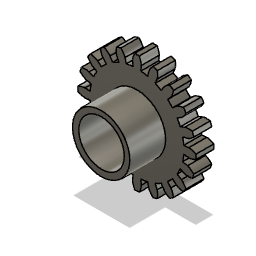
assembly (Autodesk Fusion 360 archive; units mm, degrees)
design "Small Gear(30mm)"
Autodesk Fusion 360 part; units mm, degrees
sketch "Sketch1" plane through (0, 0, 0) normal (0, 0, 1) x (1, 0, 0)
  spline S0 degree 5 poles (14.4718, -1.2197) (14.4719, -1.2197) (14.4721, -1.2197) (14.4724, -1.2198) (14.473, -1.2198) (14.4738, -1.2199) (14.4747, -1.2199) (14.4757, -1.22) (14.4769, -1.22) (14.4781, -1.2201) (14.4795, -1.2202) (14.481, -1.2203) (14.4826, -1.2203) (14.4844, -1.2204) (14.4862, -1.2205) (14.4881, -1.2205) (14.4902, -1.2206) (14.4923, -1.2207) (14.4946, -1.2207) (14.497, -1.2208) (14.4994, -1.2209) (14.502, -1.2209) (14.5047, -1.221) (14.5074, -1.221) (14.5103, -1.221) (14.5133, -1.2211) (14.5163, -1.2211) (14.5195, -1.2211) (14.5227, -1.2211) (14.5261, -1.2211) (14.5295, -1.2211) (14.533, -1.2211) (14.5366, -1.221) (14.5403, -1.221) (14.5441, -1.2209) (14.548, -1.2208) (14.5519, -1.2208) (14.556, -1.2207) (14.5601, -1.2206) (14.5643, -1.2204) (14.5686, -1.2203) (14.573, -1.2202) (14.5775, -1.22) (14.582, -1.2198) (14.5866, -1.2196) (14.5913, -1.2194) (14.5961, -1.2192) (14.601, -1.219) (14.6059, -1.2187) (14.6109, -1.2185) (14.616, -1.2182) (14.6212, -1.2179) (14.6264, -1.2176) (14.6317, -1.2172) (14.6371, -1.2169) (14.6425, -1.2165) (14.648, -1.2161) (14.6536, -1.2157) (14.6593, -1.2153) (14.665, -1.2148) (14.6708, -1.2143) (14.6767, -1.2139) (14.6827, -1.2133) (14.6887, -1.2128) (14.6947, -1.2123) (14.7009, -1.2117) (14.7071, -1.2111) (14.7133, -1.2105) (14.7197, -1.2098) (14.7261, -1.2092) (14.7325, -1.2085) (14.7391, -1.2078) (14.7457, -1.2071) (14.7523, -1.2063) (14.759, -1.2056) (14.7658, -1.2048) (14.7726, -1.204) (14.7795, -1.2031) (14.7865, -1.2023) (14.7935, -1.2014) (14.8006, -1.2005) (14.8077, -1.1995) (14.8149, -1.1986) (14.8221, -1.1976) (14.8294, -1.1966) (14.8368, -1.1955) (14.8442, -1.1945) (14.8517, -1.1934) (14.8592, -1.1923) (14.8668, -1.1911) (14.8744, -1.19) (14.8821, -1.1888) (14.8899, -1.1876) (14.8977, -1.1863) (14.9055, -1.1851) (14.9134, -1.1838) (14.9214, -1.1825) (14.9294, -1.1811) (14.9375, -1.1797) (14.9456, -1.1783) (14.9537, -1.1769) (14.9619, -1.1754) (14.9702, -1.174) (14.9785, -1.1724) (14.9869, -1.1709) (14.9953, -1.1693) (15.0037, -1.1677) (15.0122, -1.1661) (15.0208, -1.1645) (15.0294, -1.1628) (15.038, -1.1611) (15.0467, -1.1593) (15.0555, -1.1576) (15.0643, -1.1558) (15.0731, -1.1539) (15.082, -1.1521) (15.0909, -1.1502) (15.0999, -1.1483) (15.1089, -1.1463) (15.1179, -1.1444) (15.127, -1.1423) (15.1362, -1.1403) (15.1454, -1.1382) (15.1546, -1.1361) (15.1639, -1.134) (15.1732, -1.1319) (15.1825, -1.1297) (15.1919, -1.1275) (15.2014, -1.1252) (15.2109, -1.1229) (15.2204, -1.1206) (15.2299, -1.1183) (15.2395, -1.1159) (15.2492, -1.1135) (15.2589, -1.1111) (15.2686, -1.1086) (15.2783, -1.1061) (15.2881, -1.1036) (15.298, -1.101) (15.3079, -1.0984) (15.3178, -1.0958) (15.3277, -1.0931) (15.3377, -1.0905) (15.3477, -1.0877) (15.3578, -1.085) (15.3679, -1.0822) (15.3781, -1.0794) (15.3882, -1.0765) (15.3984, -1.0737) (15.4087, -1.0707) (15.419, -1.0678) (15.4293, -1.0648) (15.4396, -1.0618) (15.45, -1.0587) (15.4604, -1.0557) (15.4709, -1.0526) (15.4814, -1.0494) (15.4919, -1.0462) (15.5025, -1.043) (15.513, -1.0398) (15.5237, -1.0365) (15.5343, -1.0332) (15.545, -1.0298) (15.5557, -1.0265) (15.5665, -1.0231) (15.5773, -1.0196) (15.5881, -1.0161) (15.5989, -1.0126) (15.6098, -1.0091) (15.6207, -1.0055) (15.6317, -1.0019) (15.6426, -0.9982) (15.6536, -0.9945) (15.6647, -0.9908) (15.6757, -0.9871) (15.6868, -0.9833) (15.6979, -0.9795) (15.7091, -0.9756) (15.7203, -0.9717) (15.7315, -0.9678) (15.7427, -0.9638) (15.754, -0.9598) (15.7653, -0.9558) (15.7766, -0.9518) (15.7879, -0.9477) (15.7993, -0.9435) (15.8107, -0.9394) (15.8222, -0.9352) (15.8336, -0.9309) (15.8451, -0.9267) (15.8566, -0.9223) (15.8681, -0.918) (15.8797, -0.9136) (15.8913, -0.9092) (15.9029, -0.9048) (15.9146, -0.9003) (15.9262, -0.8958) (15.9379, -0.8912) (15.9496, -0.8866) (15.9614, -0.882) (15.9731, -0.8773) (15.9849, -0.8727) (15.9967, -0.8679) (16.0086, -0.8632) (16.0205, -0.8584) (16.0323, -0.8535) (16.0442, -0.8487) (16.0562, -0.8437) (16.0681, -0.8388) (16.0801, -0.8338) (16.0921, -0.8288) (16.1041, -0.8238) (16.1162, -0.8187) (16.1283, -0.8135) (16.1404, -0.8084) (16.1525, -0.8032) (16.1646, -0.798) (16.1768, -0.7927) (16.1889, -0.7874) (16.2011, -0.7821) (16.2134, -0.7767) (16.2256, -0.7713) (16.2379, -0.7658) (16.2502, -0.7603) (16.2625, -0.7548) (16.2748, -0.7493) (16.2871, -0.7437) (16.2995, -0.738) (16.3119, -0.7324) (16.3243, -0.7267) (16.3367, -0.7209) (16.3491, -0.7152) (16.3616, -0.7094) (16.3741, -0.7035) (16.3866, -0.6976) (16.3991, -0.6917) (16.4116, -0.6858) (16.4242, -0.6798) (16.4368, -0.6737) (16.4493, -0.6677) (16.4619, -0.6616) (16.472, -0.6567) (16.4796, -0.653) (16.4847, -0.6505) (16.4872, -0.6492) knots 0 0 0 0 0 0 0.00416667 0.00833333 0.0125 0.01666667 0.02083333 0.025 0.02916667 0.03333333 0.0375 0.04166667 0.04583333 0.05 0.05416667 0.05833333 0.0625 0.06666667 0.07083333 0.075 0.07916667 0.08333333 0.0875 0.09166667 0.09583333 0.1 0.10416667 0.10833333 0.1125 0.11666667 0.12083333 0.125 0.12916667 0.13333333 0.1375 0.14166667 0.14583333 0.15 0.15416667 0.15833333 0.1625 0.16666667 0.17083333 0.175 0.17916667 0.18333333 0.1875 0.19166667 0.19583333 0.2 0.20416667 0.20833333 0.2125 0.21666667 0.22083333 0.225 0.22916667 0.23333333 0.2375 0.24166667 0.24583333 0.25 0.25416667 0.25833333 0.2625 0.26666667 0.27083333 0.275 0.27916667 0.28333333 0.2875 0.29166667 0.29583333 0.3 0.30416667 0.30833333 0.3125 0.31666667 0.32083333 0.325 0.32916667 0.33333333 0.3375 0.34166667 0.34583333 0.35 0.35416667 0.35833333 0.3625 0.36666667 0.37083333 0.375 0.37916667 0.38333333 0.3875 0.39166667 0.39583333 0.4 0.40416667 0.40833333 0.4125 0.41666667 0.42083333 0.425 0.42916667 0.43333333 0.4375 0.44166667 0.44583333 0.45 0.45416667 0.45833333 0.4625 0.46666667 0.47083333 0.475 0.47916667 0.48333333 0.4875 0.49166667 0.49583333 0.5 0.50416667 0.50833333 0.5125 0.51666667 0.52083333 0.525 0.52916667 0.53333333 0.5375 0.54166667 0.54583333 0.55 0.55416667 0.55833333 0.5625 0.56666667 0.57083333 0.575 0.57916667 0.58333333 0.5875 0.59166667 0.59583333 0.6 0.60416667 0.60833333 0.6125 0.61666667 0.62083333 0.625 0.62916667 0.63333333 0.6375 0.64166667 0.64583333 0.65 0.65416667 0.65833333 0.6625 0.66666667 0.67083333 0.675 0.67916667 0.68333333 0.6875 0.69166667 0.69583333 0.7 0.70416667 0.70833333 0.7125 0.71666667 0.72083333 0.725 0.72916667 0.73333333 0.7375 0.74166667 0.74583333 0.75 0.75416667 0.75833333 0.7625 0.76666667 0.77083333 0.775 0.77916667 0.78333333 0.7875 0.79166667 0.79583333 0.8 0.80416667 0.80833333 0.8125 0.81666667 0.82083333 0.825 0.82916667 0.83333333 0.8375 0.84166667 0.84583333 0.85 0.85416667 0.85833333 0.8625 0.86666667 0.87083333 0.875 0.87916667 0.88333333 0.8875 0.89166667 0.89583333 0.9 0.90416667 0.90833333 0.9125 0.91666667 0.92083333 0.925 0.92916667 0.93333333 0.9375 0.94166667 0.94583333 0.95 0.95416667 0.95833333 0.9625 0.96666667 0.97083333 0.975 0.97916667 0.98333333 0.9875 0.99166667 0.99583333 1 1 1 1 1 1
  spline S1 degree 5 poles (14.4718, 1.2197) (14.4719, 1.2197) (14.4721, 1.2197) (14.4724, 1.2198) (14.473, 1.2198) (14.4738, 1.2199) (14.4747, 1.2199) (14.4757, 1.22) (14.4769, 1.22) (14.4781, 1.2201) (14.4795, 1.2202) (14.481, 1.2203) (14.4826, 1.2203) (14.4844, 1.2204) (14.4862, 1.2205) (14.4881, 1.2205) (14.4902, 1.2206) (14.4923, 1.2207) (14.4946, 1.2207) (14.497, 1.2208) (14.4994, 1.2209) (14.502, 1.2209) (14.5047, 1.221) (14.5074, 1.221) (14.5103, 1.221) (14.5133, 1.2211) (14.5163, 1.2211) (14.5195, 1.2211) (14.5227, 1.2211) (14.5261, 1.2211) (14.5295, 1.2211) (14.533, 1.2211) (14.5366, 1.221) (14.5403, 1.221) (14.5441, 1.2209) (14.548, 1.2208) (14.5519, 1.2208) (14.556, 1.2207) (14.5601, 1.2206) (14.5643, 1.2204) (14.5686, 1.2203) (14.573, 1.2202) (14.5775, 1.22) (14.582, 1.2198) (14.5866, 1.2196) (14.5913, 1.2194) (14.5961, 1.2192) (14.601, 1.219) (14.6059, 1.2187) (14.6109, 1.2185) (14.616, 1.2182) (14.6212, 1.2179) (14.6264, 1.2176) (14.6317, 1.2172) (14.6371, 1.2169) (14.6425, 1.2165) (14.648, 1.2161) (14.6536, 1.2157) (14.6593, 1.2153) (14.665, 1.2148) (14.6708, 1.2143) (14.6767, 1.2139) (14.6827, 1.2133) (14.6887, 1.2128) (14.6947, 1.2123) (14.7009, 1.2117) (14.7071, 1.2111) (14.7133, 1.2105) (14.7197, 1.2098) (14.7261, 1.2092) (14.7325, 1.2085) (14.7391, 1.2078) (14.7457, 1.2071) (14.7523, 1.2063) (14.759, 1.2056) (14.7658, 1.2048) (14.7726, 1.204) (14.7795, 1.2031) (14.7865, 1.2023) (14.7935, 1.2014) (14.8006, 1.2005) (14.8077, 1.1995) (14.8149, 1.1986) (14.8221, 1.1976) (14.8294, 1.1966) (14.8368, 1.1955) (14.8442, 1.1945) (14.8517, 1.1934) (14.8592, 1.1923) (14.8668, 1.1911) (14.8744, 1.19) (14.8821, 1.1888) (14.8899, 1.1876) (14.8977, 1.1863) (14.9055, 1.1851) (14.9134, 1.1838) (14.9214, 1.1825) (14.9294, 1.1811) (14.9375, 1.1797) (14.9456, 1.1783) (14.9537, 1.1769) (14.9619, 1.1754) (14.9702, 1.174) (14.9785, 1.1724) (14.9869, 1.1709) (14.9953, 1.1693) (15.0037, 1.1677) (15.0122, 1.1661) (15.0208, 1.1645) (15.0294, 1.1628) (15.038, 1.1611) (15.0467, 1.1593) (15.0555, 1.1576) (15.0643, 1.1558) (15.0731, 1.1539) (15.082, 1.1521) (15.0909, 1.1502) (15.0999, 1.1483) (15.1089, 1.1463) (15.1179, 1.1444) (15.127, 1.1423) (15.1362, 1.1403) (15.1454, 1.1382) (15.1546, 1.1361) (15.1639, 1.134) (15.1732, 1.1319) (15.1825, 1.1297) (15.1919, 1.1275) (15.2014, 1.1252) (15.2109, 1.1229) (15.2204, 1.1206) (15.2299, 1.1183) (15.2395, 1.1159) (15.2492, 1.1135) (15.2589, 1.1111) (15.2686, 1.1086) (15.2783, 1.1061) (15.2881, 1.1036) (15.298, 1.101) (15.3079, 1.0984) (15.3178, 1.0958) (15.3277, 1.0931) (15.3377, 1.0905) (15.3477, 1.0877) (15.3578, 1.085) (15.3679, 1.0822) (15.3781, 1.0794) (15.3882, 1.0765) (15.3984, 1.0737) (15.4087, 1.0707) (15.419, 1.0678) (15.4293, 1.0648) (15.4396, 1.0618) (15.45, 1.0587) (15.4604, 1.0557) (15.4709, 1.0526) (15.4814, 1.0494) (15.4919, 1.0462) (15.5025, 1.043) (15.513, 1.0398) (15.5237, 1.0365) (15.5343, 1.0332) (15.545, 1.0298) (15.5557, 1.0265) (15.5665, 1.0231) (15.5773, 1.0196) (15.5881, 1.0161) (15.5989, 1.0126) (15.6098, 1.0091) (15.6207, 1.0055) (15.6317, 1.0019) (15.6426, 0.9982) (15.6536, 0.9945) (15.6647, 0.9908) (15.6757, 0.9871) (15.6868, 0.9833) (15.6979, 0.9795) (15.7091, 0.9756) (15.7203, 0.9717) (15.7315, 0.9678) (15.7427, 0.9638) (15.754, 0.9598) (15.7653, 0.9558) (15.7766, 0.9518) (15.7879, 0.9477) (15.7993, 0.9435) (15.8107, 0.9394) (15.8222, 0.9352) (15.8336, 0.9309) (15.8451, 0.9267) (15.8566, 0.9223) (15.8681, 0.918) (15.8797, 0.9136) (15.8913, 0.9092) (15.9029, 0.9048) (15.9146, 0.9003) (15.9262, 0.8958) (15.9379, 0.8912) (15.9496, 0.8866) (15.9614, 0.882) (15.9731, 0.8773) (15.9849, 0.8727) (15.9967, 0.8679) (16.0086, 0.8632) (16.0205, 0.8584) (16.0323, 0.8535) (16.0442, 0.8487) (16.0562, 0.8437) (16.0681, 0.8388) (16.0801, 0.8338) (16.0921, 0.8288) (16.1041, 0.8238) (16.1162, 0.8187) (16.1283, 0.8135) (16.1404, 0.8084) (16.1525, 0.8032) (16.1646, 0.798) (16.1768, 0.7927) (16.1889, 0.7874) (16.2011, 0.7821) (16.2134, 0.7767) (16.2256, 0.7713) (16.2379, 0.7658) (16.2502, 0.7603) (16.2625, 0.7548) (16.2748, 0.7493) (16.2871, 0.7437) (16.2995, 0.738) (16.3119, 0.7324) (16.3243, 0.7267) (16.3367, 0.7209) (16.3491, 0.7152) (16.3616, 0.7094) (16.3741, 0.7035) (16.3866, 0.6976) (16.3991, 0.6917) (16.4116, 0.6858) (16.4242, 0.6798) (16.4368, 0.6737) (16.4493, 0.6677) (16.4619, 0.6616) (16.472, 0.6567) (16.4796, 0.653) (16.4847, 0.6505) (16.4872, 0.6492) knots 0 0 0 0 0 0 0.00416667 0.00833333 0.0125 0.01666667 0.02083333 0.025 0.02916667 0.03333333 0.0375 0.04166667 0.04583333 0.05 0.05416667 0.05833333 0.0625 0.06666667 0.07083333 0.075 0.07916667 0.08333333 0.0875 0.09166667 0.09583333 0.1 0.10416667 0.10833333 0.1125 0.11666667 0.12083333 0.125 0.12916667 0.13333333 0.1375 0.14166667 0.14583333 0.15 0.15416667 0.15833333 0.1625 0.16666667 0.17083333 0.175 0.17916667 0.18333333 0.1875 0.19166667 0.19583333 0.2 0.20416667 0.20833333 0.2125 0.21666667 0.22083333 0.225 0.22916667 0.23333333 0.2375 0.24166667 0.24583333 0.25 0.25416667 0.25833333 0.2625 0.26666667 0.27083333 0.275 0.27916667 0.28333333 0.2875 0.29166667 0.29583333 0.3 0.30416667 0.30833333 0.3125 0.31666667 0.32083333 0.325 0.32916667 0.33333333 0.3375 0.34166667 0.34583333 0.35 0.35416667 0.35833333 0.3625 0.36666667 0.37083333 0.375 0.37916667 0.38333333 0.3875 0.39166667 0.39583333 0.4 0.40416667 0.40833333 0.4125 0.41666667 0.42083333 0.425 0.42916667 0.43333333 0.4375 0.44166667 0.44583333 0.45 0.45416667 0.45833333 0.4625 0.46666667 0.47083333 0.475 0.47916667 0.48333333 0.4875 0.49166667 0.49583333 0.5 0.50416667 0.50833333 0.5125 0.51666667 0.52083333 0.525 0.52916667 0.53333333 0.5375 0.54166667 0.54583333 0.55 0.55416667 0.55833333 0.5625 0.56666667 0.57083333 0.575 0.57916667 0.58333333 0.5875 0.59166667 0.59583333 0.6 0.60416667 0.60833333 0.6125 0.61666667 0.62083333 0.625 0.62916667 0.63333333 0.6375 0.64166667 0.64583333 0.65 0.65416667 0.65833333 0.6625 0.66666667 0.67083333 0.675 0.67916667 0.68333333 0.6875 0.69166667 0.69583333 0.7 0.70416667 0.70833333 0.7125 0.71666667 0.72083333 0.725 0.72916667 0.73333333 0.7375 0.74166667 0.74583333 0.75 0.75416667 0.75833333 0.7625 0.76666667 0.77083333 0.775 0.77916667 0.78333333 0.7875 0.79166667 0.79583333 0.8 0.80416667 0.80833333 0.8125 0.81666667 0.82083333 0.825 0.82916667 0.83333333 0.8375 0.84166667 0.84583333 0.85 0.85416667 0.85833333 0.8625 0.86666667 0.87083333 0.875 0.87916667 0.88333333 0.8875 0.89166667 0.89583333 0.9 0.90416667 0.90833333 0.9125 0.91666667 0.92083333 0.925 0.92916667 0.93333333 0.9375 0.94166667 0.94583333 0.95 0.95416667 0.95833333 0.9625 0.96666667 0.97083333 0.975 0.97916667 0.98333333 0.9875 0.99166667 0.99583333 1 1 1 1 1 1
  spline S2 degree 5 poles (14.4709, -1.2197) (14.4709, -1.2197) (14.471, -1.2197) (14.4711, -1.2197) (14.4713, -1.2197) (14.4714, -1.2197) (14.4716, -1.2197) (14.4717, -1.2197) (14.4717, -1.2197) (14.4718, -1.2197) knots 0 0 0 0 0 0 0.2 0.4 0.6 0.8 1 1 1 1 1 1
  spline S3 degree 5 poles (14.4709, 1.2197) (14.4709, 1.2197) (14.471, 1.2197) (14.4711, 1.2197) (14.4713, 1.2197) (14.4714, 1.2197) (14.4716, 1.2197) (14.4717, 1.2197) (14.4717, 1.2197) (14.4718, 1.2197) knots 0 0 0 0 0 0 0.2 0.4 0.6 0.8 1 1 1 1 1 1
  line L0 (0, 0) -> (14.4709, -1.2197)
  line L1 (0, 0) -> (14.4709, 1.2197)
  arc A0 (16.4872, -0.6492) -> (16.4872, 0.6492) centre (0, 0) ccw
  point P0 (14.4744, -1.2199)
  point P1 (14.4788, -1.2201)
  point P2 (14.485, -1.2204)
  point P3 (14.4929, -1.2207)
  point P4 (14.5026, -1.2209)
  point P5 (14.514, -1.2211)
  point P6 (14.5272, -1.2211)
  point P7 (14.5421, -1.2209)
  point P8 (14.5589, -1.2206)
  point P9 (14.5773, -1.22)
  point P10 (14.5975, -1.2192)
  point P11 (14.6195, -1.218)
  point P12 (14.6432, -1.2164)
  point P13 (14.6687, -1.2145)
  point P14 (14.6958, -1.2122)
  point P15 (14.7247, -1.2093)
  point P16 (14.7553, -1.206)
  point P17 (14.7877, -1.2021)
  point P18 (14.8217, -1.1976)
  point P19 (14.8574, -1.1925)
  point P20 (14.8948, -1.1868)
  point P21 (14.9338, -1.1803)
  point P22 (14.9746, -1.1732)
  point P23 (15.0169, -1.1652)
  point P24 (15.0609, -1.1564)
  point P25 (15.1066, -1.1468)
  point P26 (15.1538, -1.1363)
  point P27 (15.2026, -1.1249)
  point P28 (15.2531, -1.1125)
  point P29 (15.305, -1.0992)
  point P30 (15.3586, -1.0848)
  point P31 (15.4136, -1.0693)
  point P32 (15.4702, -1.0528)
  point P33 (15.5283, -1.0351)
  point P34 (15.5878, -1.0162)
  point P35 (15.6488, -0.9961)
  point P36 (15.7113, -0.9748)
  point P37 (15.7752, -0.9523)
  point P38 (15.8404, -0.9284)
  point P39 (15.9071, -0.9032)
  point P40 (15.9751, -0.8766)
  point P41 (16.0444, -0.8486)
  point P42 (16.1151, -0.8191)
  point P43 (16.187, -0.7882)
  point P44 (16.2603, -0.7558)
  point P45 (16.3347, -0.7219)
  point P46 (16.4104, -0.6863)
  point P47 (14.4744, 1.2199)
  point P48 (14.4788, 1.2201)
  point P49 (14.485, 1.2204)
  point P50 (14.4929, 1.2207)
  point P51 (14.5026, 1.2209)
  point P52 (14.514, 1.2211)
  point P53 (14.5272, 1.2211)
  point P54 (14.5421, 1.2209)
  point P55 (14.5589, 1.2206)
  point P56 (14.5773, 1.22)
  point P57 (14.5975, 1.2192)
  point P58 (14.6195, 1.218)
  point P59 (14.6432, 1.2164)
  point P60 (14.6687, 1.2145)
  point P61 (14.6958, 1.2122)
  point P62 (14.7247, 1.2093)
  point P63 (14.7553, 1.206)
  point P64 (14.7877, 1.2021)
  point P65 (14.8217, 1.1976)
  point P66 (14.8574, 1.1925)
  point P67 (14.8948, 1.1868)
  point P68 (14.9338, 1.1803)
  point P69 (14.9746, 1.1732)
  point P70 (15.0169, 1.1652)
  point P71 (15.0609, 1.1564)
  point P72 (15.1066, 1.1468)
  point P73 (15.1538, 1.1363)
  point P74 (15.2026, 1.1249)
  point P75 (15.2531, 1.1125)
  point P76 (15.305, 1.0992)
  point P77 (15.3586, 1.0848)
  point P78 (15.4136, 1.0693)
  point P79 (15.4702, 1.0528)
  point P80 (15.5283, 1.0351)
  point P81 (15.5878, 1.0162)
  point P82 (15.6488, 0.9961)
  point P83 (15.7113, 0.9748)
  point P84 (15.7752, 0.9523)
  point P85 (15.8404, 0.9284)
  point P86 (15.9071, 0.9032)
  point P87 (15.9751, 0.8766)
  point P88 (16.0444, 0.8486)
  point P89 (16.1151, 0.8191)
  point P90 (16.187, 0.7882)
  point P91 (16.2603, 0.7558)
  point P92 (16.3347, 0.7219)
  point P93 (16.4104, 0.6863)
sketch "Sketch2" plane through (0, 0, 0) normal (0, 0, 1) x (1, 0, 0)
  circle A0 centre (0, 0) radius 13.125
extrude "Extrude1" add sketch "Sketch2" along normal blind 5 makes body 1
extrude "Extrude2" add sketch "Sketch1" along normal blind 5 separate body makes body 2
pattern_circular "C-Pattern1" count 20 over 360 about axis through (0, 0, 1.75) along (0, 0, 1) of "Extrude2" makes body 3 at (4.7135, 1.104, 1.6667) makes body 4 at (4.1416, 2.5065, 1.6667) makes body 5 at (3.1644, 3.6637, 1.6667) makes body 6 at (1.8774, 4.4622, 1.6667) makes body 7 at (0.4066, 4.8239, 1.6667) makes body 8 at (-1.104, 4.7135, 1.6667) makes body 9 at (-3.1644, 3.6637, 1.6667) makes body 10 at (-3.6637, 3.1644, 1.6667) makes body 11 at (-4.7135, 1.104, 1.6667) makes body 12 at (-4.8239, 0.4066, 1.6667) makes body 13 at (-4.7135, -1.104, 1.6667) makes body 14 at (-3.6637, -3.1644, 1.6667) makes body 15 at (-3.1644, -3.6637, 1.6667) makes body 16 at (-1.8774, -4.4622, 1.6667) makes body 17 at (-0.4066, -4.8239, 1.6667) makes body 18 at (1.104, -4.7135, 1.6667) makes body 19 at (2.5065, -4.1416, 1.6667) makes body 20 at (3.6637, -3.1644, 1.6667) makes body 21 at (4.4622, -1.8774, 1.6667)
combine "Combine1" operation add target body 1 tool bodies 2 3 4 5 6 7 8 9 10 11 12 13 14 15 16 17 18 19 20 21
sketch "Sketch3" plane through (0, 0, 0) normal (0, 0, 1) x (1, 0, 0)
  line L0 (0, 0) -> (48.3003, 0) construction
  line L1 (48.3003, 0) -> (48.3003, 3) construction
  line L2 (48.3003, 3) -> (0, 3) construction
  line L3 (0, 3) -> (0, 0) construction
  constraint perpendicular L0 L1
  constraint parallel L0 L2
  constraint parallel L1 L3
cylinder "CylinderPrimitive1" add diameter 16 height 10 placed x (1, 0, 0) y (0, 1, 0) z (0, 0, 1) at (0, 0, 5) bodies 1
hole "Hole1" at (0.103, 0.1545, 15) direction (0, 0, -1) diameter 12.7 depth 30 tip angle 118 bodies 1

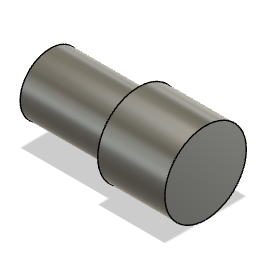
design "motor finale"
Autodesk Fusion 360 part; units mm, degrees
cylinder "CylinderPrimitive1" add diameter 37 height 30.5 placed x (0, 0, -1) y (0, 1, 0) z (1, 0, 0) at (0, 0, 0)
cylinder "CylinderPrimitive2" add diameter 27.5 height 40 placed x (0, 0, 1) y (0, 1, 0) z (-1, 0, 0) at (0, 0, 0)

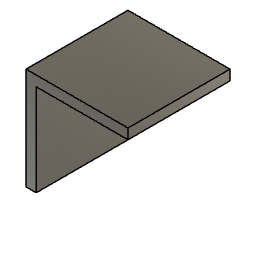
design "L_Support"
Autodesk Fusion 360 part; units mm, degrees
sketch "Sketch1" plane through (0, 0, 0) normal (0, 1, 0) x (1, 0, 0)
  line L0 (0, 0) -> (5, 0)
  line L1 (5, 0) -> (5, -50)
  line L2 (5, -50) -> (0, -50)
  line L3 (0, -50) -> (0, 0)
  line L4 (0, -50) -> (50, -50)
  line L5 (50, -50) -> (50, -45)
  line L6 (50, -45) -> (0, -45)
  line L7 (0, -45) -> (0, -50)
  dimension "d1" = 5
  dimension "d2" = 50
  dimension "d3" = 50
  dimension "d4" = 5
  constraint horizontal L0
  constraint vertical L1
  constraint horizontal L2
  constraint vertical L3
  constraint coincident L0.start L3.end
  constraint horizontal L4
  constraint vertical L5
  constraint horizontal L6
  constraint vertical L7
  measures "d1" distance of L0.start L0.end
  measures "d2" distance of L0.start L2.end
  measures "d3" distance of L2.end L4.end
  measures "d4" distance of L2.end L6.end
extrude "Extrude1" add sketch "Sketch1" along normal blind 50

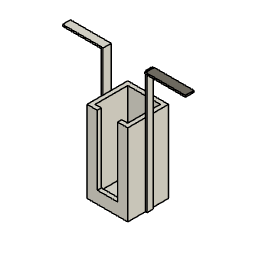
design "Container Seed"
Autodesk Fusion 360 part; units mm, degrees
sketch "Sketch1" plane through (0, 0, 0) normal (0, 0, 1) x (1, 0, 0)
  line L0 (0, 0) -> (50, 0)
  line L1 (50, 0) -> (50, 50)
  line L2 (50, 50) -> (0, 50)
  line L3 (0, 50) -> (0, 0)
  line L4 (5, 5) -> (45, 5)
  line L5 (45, 5) -> (45, 45)
  line L6 (45, 45) -> (5, 45)
  line L7 (5, 45) -> (5, 5)
  dimension "d1" = 50
  dimension "d2" = 50
  dimension "d3" = 40
  constraint horizontal L0
  constraint vertical L1
  constraint horizontal L2
  constraint vertical L3
  constraint coincident L0.start L3.end
  constraint horizontal L4
  constraint vertical L5
  constraint horizontal L6
  constraint vertical L7
  measures "d1" distance of L0.start L0.end
  measures "d2" distance of L0.start L2.end
  measures "d3" distance of L4.start L4.end
extrude "Extrude1" add sketch "Sketch1" along normal blind 95 makes body 1
sketch "Sketch2" plane through (0, 0, 0) normal (0, 0, 1) x (1, 0, 0)
  line L0 (0, 0) -> (50, 0)
  line L1 (50, 0) -> (50, 50)
  line L2 (50, 50) -> (0, 50)
  line L3 (0, 50) -> (0, 0)
  constraint horizontal L0
  constraint vertical L1
  constraint horizontal L2
  constraint vertical L3
  constraint coincident L0.start L3.end
extrude "Extrude2" add sketch "Sketch2" against normal blind 5 bodies 1
sketch "Sketch3" plane through (0, 0, 0) normal (0, 1, 0) x (1, 0, 0)
  line L0 (25, -95) -> (12.5, -95)
  line L1 (12.5, -95) -> (12.5, -30)
  line L2 (12.5, -30) -> (25, -30)
  line L3 (25, -30) -> (25, -95)
  dimension "d8" = 12.5
  dimension "d9" = 65
  constraint horizontal L0
  constraint vertical L1
  constraint horizontal L2
  constraint vertical L3
  measures "d8" distance of L0.start L0.end
  measures "d9" distance of L0.start L2.end
sketch "Sketch4" plane through (0, 0, 0) normal (0, 1, 0) x (1, 0, 0)
  line L0 (25, -30) -> (37.5, -30)
  line L1 (37.5, -30) -> (37.5, -95)
  line L2 (37.5, -95) -> (25, -95)
  line L3 (25, -95) -> (25, -30)
  dimension "d10" = 12.5
  dimension "d11" = 65
  constraint horizontal L0
  constraint vertical L1
  constraint horizontal L2
  constraint vertical L3
  measures "d10" distance of L0.start L0.end
  measures "d11" distance of L0.start L2.end
extrude "Extrude3" cut sketch "Sketch3" along normal blind 20 bodies 1
extrude "Extrude4" cut sketch "Sketch4" along normal blind 10 bodies 1
extrude "Extrude5" cut 1 faces at (20.8333, 1.6667, 30) along direction (0, 0, -1) blind 20 on bodies 1 bodies 1
box "BoxPrimitive1" add length 150 width 7.6164 height 2 placed x (0, 0, 1) y (0, -1, 0) z (1, 0, 0) at (50, 29.2955, -5) bodies 1
box "BoxPrimitive2" add length 150 width 10.3045 height 2 placed x (0, 0, 1) y (0, 1, 0) z (-1, 0, 0) at (0, 19.439, -5) bodies 1
box "BoxPrimitive3" add length 2 width 9.6811 height -50 placed x (0, 0, 1) y (0, -1, 0) z (1, 0, 0) at (0, 29.6811, 143) bodies 1
box "BoxPrimitive4" add length 2 width 10.4962 height 50 placed x (0, 0, 1) y (0, -1, 0) z (1, 0, 0) at (0, -89.5038, 150) separate body makes body 2
move_body "Move1" bodies 2 to x (1, 0, 0) y (0, 1, 0) z (0, 0, 1) at (50.5817, 120.1851, -7.2633)

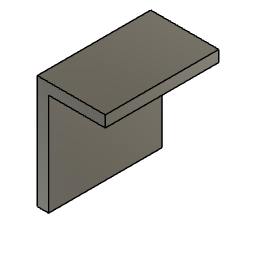
design "Motor Mount"
Autodesk Fusion 360 part; units mm, degrees
sketch "Sketch1" plane through (0, 0, 0) normal (0, 1, 0) x (1, 0, 0)
  line L0 (0, 0) -> (5, 0)
  line L1 (5, 0) -> (5, -50)
  line L2 (5, -50) -> (0, -50)
  line L3 (0, -50) -> (0, 0)
  line L4 (0, -50) -> (30, -50)
  line L5 (30, -50) -> (30, -45)
  line L6 (30, -45) -> (0, -45)
  line L7 (0, -45) -> (0, -50)
  dimension "d1" = 5
  dimension "d2" = 30
  constraint horizontal L0
  constraint vertical L1
  constraint horizontal L2
  constraint vertical L3
  constraint coincident L0.start L3.end
  constraint horizontal L4
  constraint vertical L5
  constraint horizontal L6
  constraint vertical L7
  measures "d1" distance of L0.start L0.end
  measures "d2" distance of L2.end L4.end
extrude "Extrude1" add sketch "Sketch1" along normal blind 50

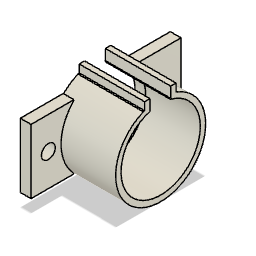
design "motor holder"
Autodesk Fusion 360 part; units mm, degrees
cylinder "CylinderPrimitive1" add diameter 42 height 30.5 placed x (0, 0, -1) y (0, 1, 0) z (1, 0, 0) at (0, 0, 0)
hole "Hole1" at (30.5, 0.1807, 0) direction (-1, 0, 0) diameter 37 depth 40 tip angle 118
hole "Hole2" at (30.5, 19.8526, 0.1413) direction (-1, 0, 0) diameter 10 depth 40 tip angle 118
fillet "Fillet1" radius 2.5 1 edges at (15.25, 20.4384, -4.8243)
fillet "Fillet2" radius 2.5 1 edges at (15.25, 20.3676, 5.1147)
box "BoxPrimitive1" add length 25 width 2.5 height 30.5 placed x (0, 1, 0) y (0, 0, 1) z (1, 0, 0) at (0, 18.1744, 5)
box "BoxPrimitive2" add length 25.1306 width 2.5 height 30.5 placed x (0, 1, 0) y (0, 0, 1) z (1, 0, 0) at (0, 18.2286, -7.2007)
extrude "Extrude1" cut 1 faces at (10.1667, 43.1744, 6.6667) along direction (0, -1, 0) blind 20
extrude "Extrude2" cut 1 faces at (10.1667, 43.3593, -5.534) along direction (0, -1, 0) blind 20
box "BoxPrimitive3" add length 30 width 20 height 5 placed x (0, -1, 0) y (0, 0, -1) z (1, 0, 0) at (0, 15, 35)
box "BoxPrimitive4" add length 30 width 20 height 5 placed x (0, -1, 0) y (0, 0, -1) z (1, 0, 0) at (0, 15, -15)
cylinder "CylinderPrimitive2" add diameter 37 height 5 placed x (0, 0, -1) y (0, 1, 0) z (1, 0, 0) at (0, 0, 0)
hole "Hole3" at (5, 0, 0) direction (-1, 0, 0) diameter 37 depth 40 tip angle 118
hole "Hole4" at (5, 0, 26.9198) direction (-1, 0, 0) diameter 6.5 depth 40 tip angle 118
hole "Hole5" at (5, 0, -25.4003) direction (-1, 0, 0) diameter 6.5 depth 40 tip angle 118

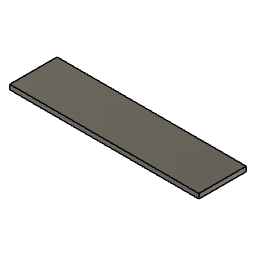
design "Flat_2"
Autodesk Fusion 360 part; units mm, degrees
sketch "Sketch1" plane through (0, 0, 0) normal (0, 0, 1) x (1, 0, 0)
  line L0 (0, 0) -> (200, 0)
  line L1 (200, 0) -> (200, 50)
  line L2 (200, 50) -> (0, 50)
  line L3 (0, 50) -> (0, 0)
  dimension "d1" = 200
  dimension "d2" = 50
  constraint horizontal L0
  constraint vertical L1
  constraint horizontal L2
  constraint vertical L3
  constraint coincident L0.start L3.end
  measures "d1" distance of L0.start L0.end
  measures "d2" distance of L0.start L2.end
extrude "Extrude1" add sketch "Sketch1" along normal blind 5

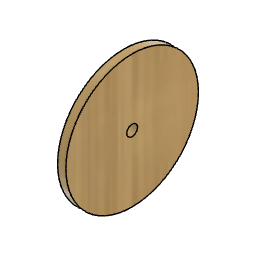
design "Wheel_"
Autodesk Fusion 360 part; units mm, degrees
sketch "Sketch1" plane through (0, 0, 0) normal (1, 0, 0) x (0, 1, 0)
  circle A0 centre (0, 0) radius 80
  dimension "d1" = 160
  constraint coincident A0.centre origin
  measures "d1" diameter of A0
extrude "Extrude1" add sketch "Sketch1" along normal blind 10
sketch "Sketch2" plane through (10, 0, 0) normal (1, 0, 0) x (0, 1, 0)
  circle A0 centre (0, 0) radius 80
  circle A1 centre (0, 0) radius 6.5
  dimension "d4" = 13
  constraint coincident A0.centre A1.centre
  measures "d4" diameter of A1
hole "Hole1" at (10, 0, 0) direction (-1, 0, 0) diameter 13 depth 30 tip angle 118

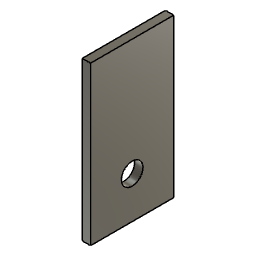
design "Flat_3"
Autodesk Fusion 360 part; units mm, degrees
sketch "Sketch1" plane through (0, 0, 0) normal (1, 0, 0) x (0, 1, 0)
  line L0 (0, 0) -> (50, 0)
  line L1 (50, 0) -> (50, 95)
  line L2 (50, 95) -> (0, 95)
  line L3 (0, 95) -> (0, 0)
  dimension "d1" = 50
  dimension "d2" = 95
  constraint horizontal L0
  constraint vertical L1
  constraint horizontal L2
  constraint vertical L3
  constraint coincident L0.start L3.end
  measures "d1" distance of L0.start L0.end
  measures "d2" distance of L0.start L2.end
extrude "Extrude1" add sketch "Sketch1" along normal blind 5
sketch "Sketch2" plane through (5, 0, 0) normal (1, 0, 0) x (0, 1, 0)
  line L0 (0, 95) -> (0, 0)
  line L1 (0, 0) -> (50, 0)
  line L2 (50, 0) -> (50, 95)
  line L3 (50, 95) -> (0, 95)
  circle A0 centre (25, 25) radius 6.5
  dimension "d5" = 13
  measures "d5" diameter of A0
hole "Hole1" at (5, 25, 25) direction (-1, 0, 0) diameter 13 depth 30 tip angle 118

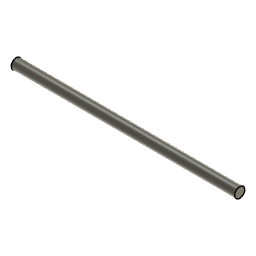
design "Axle"
Autodesk Fusion 360 part; units mm, degrees
sketch "Sketch1" plane through (0, 0, 0) normal (1, 0, 0) x (0, 1, 0)
  circle A0 centre (0, 0) radius 6.35
  dimension "d1" = 12.7
  constraint coincident A0.centre origin
  measures "d1" diameter of A0
extrude "Extrude1" add sketch "Sketch1" along normal blind 280

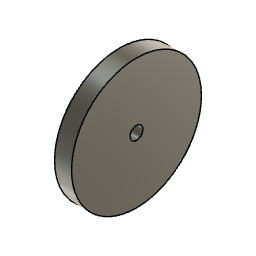
design "seed_wheel"
Autodesk Fusion 360 part; units mm, degrees
cylinder "CylinderPrimitive1" add diameter 130 height 17 placed x (0, 0, -1) y (0, 1, 0) z (1, 0, 0) at (0, 0, 0)
hole "Hole1" at (17, 0, 0) direction (-1, 0, 0) diameter 13 depth 35 tip angle 118

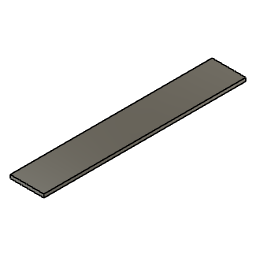
design "Flat_1"
Autodesk Fusion 360 part; units mm, degrees
sketch "Sketch1" plane through (0, 0, 0) normal (0, 0, 1) x (1, 0, 0)
  line L0 (0, 0) -> (50, 0)
  line L1 (50, 0) -> (50, 300)
  line L2 (50, 300) -> (0, 300)
  line L3 (0, 300) -> (0, 0)
  dimension "d1" = 50
  dimension "d2" = 300
  constraint horizontal L0
  constraint vertical L1
  constraint horizontal L2
  constraint vertical L3
  constraint coincident L0.start L3.end
  measures "d1" distance of L0.start L0.end
  measures "d2" distance of L0.start L2.end
extrude "Extrude1" add sketch "Sketch1" along normal blind 5
